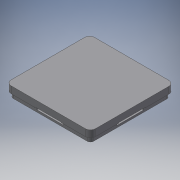
# Autodesk Inventor part: case_pantalla_3_sup
Saved by Autodesk Inventor 2019 (Build 230136000, 136)
## iProperties
Created: 2018-11-28
Part Number: case_pantalla_3_sup
Material: Steel, Mild, Welded
Document SubType Name: Modeling
Designer: cadcae
Density: 7.85 g/cm^3
Appearance: Default
Author: cadcae
Autodesk Inventor part; units mm, degrees
ref_plane "YZ Plane" through (0, 0, 0) normal (1, 0, 0) x (0, 1, 0)
ref_plane "XZ Plane" through (0, 0, 0) normal (0, 1, 0) x (-1, 0, 0)
ref_plane "XY Plane" through (0, 0, 0) normal (0, 0, 1) x (1, 0, 0)
sketch "Sketch1" plane through (0, 0, 0) normal (0, 1, 0) x (-1, 0, 0)
  line L0 (24.65, 24.4) -> (-24.65, 24.4)
  line L1 (-24.65, 24.4) -> (-24.65, -24.4)
  line L2 (-24.65, -24.4) -> (24.65, -24.4)
  line L3 (24.65, -24.4) -> (24.65, 24.4)
  line L4 (24.65, 24.4) -> (-24.65, -24.4) construction
  line L5 (-24.65, 24.4) -> (24.65, -24.4) construction
  point P0 (0, 0)
  dimension "d0" = 48.8
  dimension "d1" = 49.3
  constraints: 12 end point, 2 midpoint, 2 parallel, 1 horizontal, 1 perpendicular
  measures "d0" distance of L1.end L0.end
  measures "d1" distance of L1.end L2.end
extrude "Extrusion1" add sketch "Sketch1" along normal blind 4
fillet "Fillet1" radius 3 4 edges at (24.65, 2, 24.4) (24.65, 2, -24.4) (-24.65, 2, -24.4) (-24.65, 2, 24.4)
shell "Shell1" thickness 2.4 removed faces 1 at (7.2167, 0, -8.1333)
sketch "Sketch2" plane through (0, 0, 0) normal (0, -1, 0) x (1, 0, 0)
  arc A0 (-22.25, -21.4) -> (-21.65, -22) centre (-21.65, -21.4) ccw projected
  line L0 (-22.25, -21.4) -> (-22.25, 21.4) projected
  arc A1 (-21.65, 22) -> (-22.25, 21.4) centre (-21.65, 21.4) ccw projected
  line L1 (-21.65, 22) -> (21.65, 22) projected
  arc A2 (22.25, 21.4) -> (21.65, 22) centre (21.65, 21.4) ccw projected
  line L2 (22.25, 21.4) -> (22.25, -21.4) projected
  arc A3 (21.65, -22) -> (22.25, -21.4) centre (21.65, -21.4) ccw projected
  line L3 (21.65, -22) -> (-21.65, -22) projected
  arc A4 (-21.65, 24.4) -> (-24.65, 21.4) centre (-21.65, 21.4) ccw projected
  line L4 (-24.65, -21.4) -> (-24.65, 21.4) projected
  arc A5 (-24.65, -21.4) -> (-21.65, -24.4) centre (-21.65, -21.4) ccw projected
  line L5 (21.65, -24.4) -> (-21.65, -24.4) projected
  arc A6 (21.65, -24.4) -> (24.65, -21.4) centre (21.65, -21.4) ccw projected
  line L6 (24.65, 21.4) -> (24.65, -21.4) projected
  arc A7 (24.65, 21.4) -> (21.65, 24.4) centre (21.65, 21.4) ccw projected
  line L7 (-21.65, 24.4) -> (21.65, 24.4) projected
  line L8 (21.65, 23.2) -> (-21.65, 23.2)
  arc A8 (-21.65, 23.2) -> (-23.45, 21.4) centre (-21.65, 21.4) ccw
  line L9 (-23.45, 21.4) -> (-23.45, -21.4)
  arc A9 (-23.45, -21.4) -> (-21.65, -23.2) centre (-21.65, -21.4) ccw
  line L10 (-21.65, -23.2) -> (21.65, -23.2)
  arc A10 (21.65, -23.2) -> (23.45, -21.4) centre (21.65, -21.4) ccw
  line L11 (23.45, -21.4) -> (23.45, 21.4)
  arc A11 (23.45, 21.4) -> (21.65, 23.2) centre (21.65, 21.4) ccw
  point P0 (0, 0)
  dimension "d6" = 1.2
  constraints: 8 end point, 8 point on circle, 4 centre point, 7 other
  measures "d6" distance between parallel lines of L1 L8
extrude "Extrusion2" add sketch "Sketch2" along normal blind 3 contours A11 L11 A10 L10 A9 L9 A8 L8
sketch "Sketch5" plane through (21.65, 1.6, 22) normal (0, 0, -1) x (-1, 0, 0)
  line L0 (29.15, -3.1) -> (14.15, -3.1) projected
  line L1 (14.15, -3.1) -> (14.15, -1.6) projected
  line L2 (29.15, -1.6) -> (29.15, -3.1) projected
  line L3 (13.85, -1.6) -> (13.85, -3.4)
  line L4 (13.85, -3.4) -> (29.45, -3.4)
  line L5 (29.45, -3.4) -> (29.45, -1.6)
  line L6 (-2, -1.6) -> (0, -1.6) projected
  line L7 (43.3, -1.6) -> (0, -1.6) projected
  line L8 (13.85, -1.6) -> (29.45, -1.6)
  point P0 (21.65, -1.6)
  dimension "d10" = 0.3
  dimension "d11" = 0
  constraints: 8 end point, 1 horizontal, 2 other
  measures "d10" distance between parallel lines of L0 L4
  measures "d11" distance between parallel lines of L7 L8
extrude "Extrusion3" cut sketch "Sketch5" along normal through all both and the other way through all
sketch "Sketch6" plane through (22.25, 1.6, -21.4) normal (-1, 0, 0) x (0, 0, 1)
  line L0 (28.9, -3.1) -> (13.9, -3.1) projected
  line L1 (13.9, -3.1) -> (13.9, -1.6) projected
  line L2 (28.9, -1.6) -> (28.9, -3.1) projected
  line L3 (42.8, -1.6) -> (0, -1.6) projected
  line L4 (13.6, -1.6) -> (13.6, -3.4)
  line L5 (13.6, -3.4) -> (29.2, -3.4)
  line L6 (29.2, -3.4) -> (29.2, -1.6)
  line L7 (13.5998, -1.6) -> (29.2002, -1.6)
  point P0 (21.4, -1.6)
  dimension "d14" = 0.3
  dimension "d15" = 0.3
  dimension "d16" = 0.3
  dimension "d17" = 0
  constraints: 8 end point, 2 point on line, 1 horizontal
  measures "d14" distance between parallel lines of L0 L5
  measures "d15" distance between parallel lines of L4 L1
  measures "d16" distance between parallel lines of L2 L6
  measures "d17" distance between parallel lines of L3 L7
extrude "Extrusion4" cut sketch "Sketch6" along normal through all both and the other way through all
chamfer "Chamfer1" distance 2 angle 45 8 edges at (0, 4, -24.4) (-23.7713, 4, -23.5213) (-24.65, 4, 0) (-23.7713, 4, 23.5213) (0, 4, 24.4) (23.7713, 4, 23.5213) (24.65, 4, 0) (23.7713, 4, -23.5213)
sketch "Sketch7" plane through (-21.65, 1.6, -22) normal (0, -1, 0) x (1, 0, 0)
  line L0 (37.65, 7.5) -> (5.65, 7.5) projected
  line L1 (5.65, 7.5) -> (3.65, 7.5) projected
  arc A0 (3.65, 7.5) -> (3.65, 1) centre (3.65, 4.25) ccw projected
  line L2 (3.65, 1) -> (39.65, 1) projected
  arc A1 (39.65, 1) -> (39.65, 7.5) centre (39.65, 4.25) ccw projected
  line L3 (39.65, 7.5) -> (37.65, 7.5) projected
  circle A2 centre (3.65, 4.25) radius 1.25 projected
  circle A3 centre (39.65, 4.25) radius 1.25 construction
  line L4 (5.65, 36.5) -> (5.65, 38.5) projected
  line L5 (5.65, 38.5) -> (37.65, 38.5) projected
  line L6 (37.65, 38.5) -> (37.65, 36.5) projected
  line L7 (37.65, 36.5) -> (39.65, 36.5) projected
  arc A4 (39.65, 36.5) -> (39.65, 43) centre (39.65, 39.75) ccw projected
  line L8 (39.65, 43) -> (3.65, 43) projected
  arc A5 (3.65, 43) -> (3.65, 36.5) centre (3.65, 39.75) ccw projected
  line L9 (3.65, 36.5) -> (5.65, 36.5) projected
  circle A6 centre (3.65, 39.75) radius 1.25 projected
  circle A7 centre (39.65, 39.75) radius 1.25 construction
  line L10 (37.65, 7.5) -> (37.65, 38.5) projected
  arc A8 (39.65, 7.5) -> (39.65, 1) centre (39.65, 4.25) ccw construction
  arc A9 (39.65, 43) -> (39.65, 36.5) centre (39.65, 39.75) ccw construction
  line L11 (38.15, 1) -> (38.15, 7.5)
  line L12 (38.15, 36.5) -> (38.15, 43)
  arc A10 (39.65, 1) -> (39.65, 7.5) centre (39.65, 4.25) ccw
  arc A11 (39.65, 36.5) -> (39.65, 43) centre (39.65, 39.75) ccw
  line L13 (39.65, 1) -> (38.15, 1)
  line L14 (39.65, 7.5) -> (38.15, 7.5)
  line L15 (39.65, 36.5) -> (38.15, 36.5)
  line L16 (39.65, 43) -> (38.15, 43)
  point P0 (21.65, 22)
  dimension "d23" = 0.5
  constraints: 16 end point, 8 point on circle, 5 point on line, 4 centre point, 3 tangent, 2 coincident, 2 concentric, 2 parallel, 2 vertical, 1 collinear, 1 perpendicular, 1 other
  measures "d23" distance between parallel lines of L10 L11
extrude "Extrusion5" add sketch "Sketch7" along normal blind 5.83 contours L3 A1 L2 L11 | L8 A4 L7 L12
mirror "Mirror1" about plane through (0, 0, 0) normal (1, 0, 0) of "Extrusion5"
sketch "Sketch8" plane through (0, 4, 0) normal (0, 1, 0) x (1, 0, 0)
  circle A0 centre (0, 0) radius 5
  dimension "d26" = 10
  constraints: 1 centre point, 1 coincident
  measures "d26" diameter of A0
extrude "Extrusion6" add sketch "Sketch8" along normal blind 8.5
equation "\"d15\" = d14"
equation "\"d16\" = d14"
body "Solid1"
